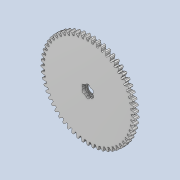
# Autodesk Inventor part: m1z57
Saved by Autodesk Inventor 2020.4 (Build 244396000, 396)
## iProperties
Created: 2021-04-23
Part Number: m1z57
Material: アルミニウム 2014-T4
Document SubType Name: Modeling
Designer: happy
Density: 2.8 g/cm^3
Appearance: サテン
Author: happy
Autodesk Inventor part; units mm, degrees
(part 1 of 2)
ref_plane "YZ Plane" through (0, 0, 0) normal (1, 0, 0) x (0, 1, 0)
ref_plane "XZ Plane" through (0, 0, 0) normal (0, 1, 0) x (-1, 0, 0)
ref_plane "XY Plane" through (0, 0, 0) normal (0, 0, 1) x (1, 0, 0)
sketch "スケッチ1" plane through (0, 0, 0) normal (0, 0, 1) x (1, 0, 0)
  arc A0 (149.0345, 132.7592) -> (148.906, 132.2471) centre (154.9871, 130.993) ccw
  arc A1 (149.29, 133.4958) -> (149.0345, 132.7592) centre (157.261, 130.3183) ccw
  arc A2 (149.7362, 134.4743) -> (149.29, 133.4958) centre (159.5861, 129.3914) ccw
  arc A3 (145.9775, 132.6493) -> (145.9061, 132.1262) centre (152.0883, 131.5486) ccw
  arc A4 (146.1504, 133.4094) -> (145.9775, 132.6493) centre (154.4226, 131.1282) ccw
  arc A5 (146.4863, 134.4312) -> (146.1504, 133.4094) centre (156.8355, 130.4627) ccw
  arc A6 (142.9512, 132.2037) -> (142.9378, 131.676) centre (149.146, 131.782) ccw
  arc A7 (143.0394, 132.9783) -> (142.9512, 132.2037) centre (151.5124, 131.6209) ccw
  arc A8 (143.2609, 134.0308) -> (143.0394, 132.9783) centre (153.9839, 131.2249) ccw
  arc A9 (139.9923, 131.428) -> (140.037, 130.9019) centre (146.1958, 131.6903) ccw
  arc A10 (139.9947, 132.2076) -> (139.9923, 131.428) centre (148.5656, 131.7905) ccw
  arc A11 (140.0991, 133.278) -> (139.9947, 132.2076) centre (151.0656, 131.6688) ccw
  arc A12 (137.1366, 130.3314) -> (137.2389, 129.8135) centre (143.2737, 131.2746) ccw
  arc A13 (137.0533, 131.1065) -> (137.1366, 130.3314) centre (145.618, 131.6349) ccw
  arc A14 (137.0393, 132.182) -> (137.0533, 131.1065) centre (148.1163, 131.789) ccw
  arc A15 (134.4189, 128.9274) -> (134.5776, 128.4239) centre (140.415, 130.5399) ccw
  arc A16 (134.2509, 129.6886) -> (134.4189, 128.9274) centre (142.7055, 131.1559) ccw
  arc A17 (134.1186, 130.756) -> (134.2509, 129.6886) centre (145.1716, 131.5839) ccw
  arc A18 (131.8722, 127.2329) -> (132.0853, 126.7499) centre (137.6545, 129.4953) ccw
  arc A19 (131.6214, 127.971) -> (131.8722, 127.2329) centre (139.8633, 130.3595) ccw
  arc A20 (131.3725, 129.0174) -> (131.6214, 127.971) centre (142.2674, 131.0562) ccw
  arc A21 (129.5273, 125.2685) -> (129.7923, 124.8119) centre (135.0256, 128.1533) ccw
  arc A22 (129.1969, 125.9746) -> (129.5273, 125.2685) centre (137.126, 129.2552) ccw
  arc A23 (128.8344, 126.9872) -> (129.1969, 125.9746) centre (139.4388, 130.2122) ccw
  arc A24 (127.4128, 123.0581) -> (127.7264, 122.6334) centre (132.5604, 126.5302) ccw
  arc A25 (127.0067, 123.7236) -> (127.4128, 123.0581) centre (134.5267, 127.8566) ccw
  arc A26 (126.535, 124.6902) -> (127.0067, 123.7236) centre (136.7203, 129.0621) ccw
  arc A27 (125.5543, 120.6285) -> (125.9126, 120.2409) centre (130.2886, 124.6458) ccw
  arc A28 (125.0774, 121.2453) -> (125.5543, 120.6285) centre (132.0972, 126.1804) ccw
  arc A29 (124.5022, 122.1541) -> (125.0774, 121.2453) centre (134.1448, 127.62) ccw
  arc A30 (123.9743, 118.0092) -> (124.3731, 117.6634) centre (128.238, 122.523) ccw
  arc A31 (123.4325, 118.5698) -> (123.9743, 118.0092) centre (129.8667, 124.2472) ccw
  arc A32 (122.7608, 119.4098) -> (123.4325, 118.5698) centre (131.7435, 125.9033) ccw
  arc A33 (122.692, 115.232) -> (123.1265, 114.9321) centre (126.4333, 120.1874) ccw
  arc A34 (122.0918, 115.7295) -> (122.692, 115.232) centre (127.8625, 122.0803) ccw
  arc A35 (121.3318, 116.4906) -> (122.0918, 115.7295) centre (129.5457, 123.9328) ccw
  arc A36 (121.7231, 112.3306) -> (122.1879, 112.0803) centre (124.8965, 117.6675) ccw
  arc A37 (121.0718, 112.7591) -> (121.7231, 112.3306) centre (126.1087, 119.7061) ccw
  arc A38 (120.2327, 113.4319) -> (121.0718, 112.7591) centre (127.578, 121.7326) ccw
  arc A39 (121.0792, 109.3402) -> (121.5687, 109.1426) centre (123.6463, 114.9938) ccw
  arc A40 (120.3847, 109.6944) -> (121.0792, 109.3402) centre (124.6269, 117.1534) ccw
  arc A41 (119.4767, 110.2709) -> (120.3847, 109.6944) centre (125.8643, 119.3292) ccw
  arc A42 (120.7682, 106.2971) -> (121.2765, 106.1545) centre (122.6977, 112.1988) ccw
  arc A43 (120.0389, 106.5728) -> (120.7682, 106.2971) centre (123.4348, 114.4532) ccw
  arc A44 (119.073, 107.0458) -> (120.0389, 106.5728) centre (124.4253, 116.7519) ccw
  arc A45 (120.7938, 103.2383) -> (121.3147, 103.1525) centre (122.0624, 109.3164) ccw
  arc A46 (120.0387, 103.4321) -> (120.7938, 103.2383) centre (122.547, 111.6382) ccw
  arc A47 (119.0266, 103.796) -> (120.0387, 103.4321) centre (123.2787, 114.0319) ccw
  arc A48 (121.1558, 100.2008) -> (121.683, 100.1728) centre (121.748, 106.3816) ccw
  arc A49 (120.3839, 100.3104) -> (121.1558, 100.2008) centre (121.9743, 108.7427) ccw
  arc A50 (119.3379, 100.5607) -> (120.3839, 100.3104) centre (122.4382, 111.2023) ccw
  arc A51 (121.8497, 97.2216) -> (122.3768, 97.2518) centre (121.7584, 103.4301) ccw
  arc A52 (121.0705, 97.2456) -> (121.8497, 97.2216) centre (121.7236, 105.8017) ccw
  arc A53 (120.0033, 97.3794) -> (121.0705, 97.2456) centre (121.9141, 108.2974) ccw
  arc A54 (122.8671, 94.3369) -> (123.3877, 94.4248) centre (122.0935, 100.4976) ccw
  arc A55 (122.09, 94.2749) -> (122.8671, 94.3369) centre (121.7979, 102.8509) ccw
  arc A56 (121.0146, 94.2905) -> (122.09, 94.2749) centre (121.7127, 105.3525) ccw
  arc A57 (124.1958, 91.5815) -> (124.7035, 91.7262) centre (122.749, 97.6197) ccw
  arc A58 (123.4302, 91.4345) -> (124.1958, 91.5815) centre (122.1964, 99.9263) ccw
  arc A59 (122.3596, 91.3317) -> (123.4302, 91.4345) centre (121.8365, 102.4033) ccw
  arc A60 (125.8194, 88.9891) -> (126.3081, 89.1888) centre (123.7172, 94.8315) ccw
  arc A61 (125.0747, 88.7587) -> (125.8194, 88.9891) centre (122.9142, 97.0633) ccw
  arc A62 (124.0219, 88.5387) -> (125.0747, 88.7587) centre (122.284, 99.4856) ccw
  arc A63 (127.7184, 86.591) -> (128.1822, 86.8432) centre (124.9863, 92.1667) ccw
  arc A64 (127.0035, 86.2801) -> (127.7184, 86.591) centre (123.9426, 94.2965) ccw
  arc A65 (125.9813, 85.9456) -> (127.0035, 86.2801) centre (123.0498, 96.6349) ccw
  arc A66 (129.8697, 84.4163) -> (130.3029, 84.7181) centre (126.5408, 89.6576) ccw
  arc A67 (129.1933, 84.0287) -> (129.8697, 84.4163) centre (125.2691, 91.6598) ccw
  arc A68 (128.2141, 83.5838) -> (129.1933, 84.0287) centre (124.1245, 93.8857) ccw
  arc A69 (132.2472, 82.4915) -> (132.6446, 82.8391) centre (128.3619, 87.3348) ccw
  arc A70 (131.6176, 82.0318) -> (132.2472, 82.4915) centre (126.8777, 89.1849) ccw
  arc A71 (130.6932, 81.4819) -> (131.6176, 82.0318) centre (125.4951, 91.2714) ccw
  arc A72 (134.822, 80.84) -> (135.1787, 81.2291) centre (130.4274, 85.2264) ccw
  arc A73 (134.2467, 80.3138) -> (134.822, 80.84) centre (128.7487, 86.902) ccw
  arc A74 (133.3885, 79.6656) -> (134.2467, 80.3138) centre (127.145, 88.8238) ccw
  arc A75 (137.5628, 79.4817) -> (137.8746, 79.9077) centre (132.7124, 83.3581) ccw
  arc A76 (137.0489, 78.8954) -> (137.5628, 79.4817) centre (130.8595, 84.8389) ccw
  arc A77 (136.2672, 78.1567) -> (137.0489, 78.8954) centre (129.0541, 86.5725) ccw
  arc A78 (140.4364, 78.4331) -> (140.6994, 78.8909) centre (135.189, 81.7524) ccw
  arc A79 (139.9902, 77.7939) -> (140.4364, 78.4331) centre (133.1845, 83.0204) ccw
  arc A80 (139.2945, 76.9737) -> (139.9902, 77.7939) centre (131.1993, 84.5449) ccw
  arc A81 (143.4079, 77.7071) -> (143.619, 78.191) centre (137.8272, 80.429) ccw
  arc A82 (143.0347, 77.0227) -> (143.4079, 77.7071) centre (135.6954, 81.4687) ccw
  arc A83 (142.4335, 76.1309) -> (143.0347, 77.0227) centre (133.5546, 82.7656) ccw
  arc A84 (146.4413, 77.3123) -> (146.5978, 77.8165) centre (140.595, 79.4038) ccw
  arc A85 (146.1456, 76.591) -> (146.4413, 77.3123) centre (138.3618, 80.2027) ccw
  arc A86 (145.6462, 75.6385) -> (146.1456, 76.591) centre (136.0913, 81.2562) ccw
  arc A87 (149.4997, 77.2537) -> (149.5998, 77.772) centre (143.4588, 78.6893) ccw
  arc A88 (149.2852, 76.5042) -> (149.4997, 77.2537) centre (141.1512, 79.2377) ccw
  arc A89 (148.8935, 75.5025) -> (149.2852, 76.5042) centre (138.7786, 80.035) ccw
  arc A90 (152.546, 77.5318) -> (152.5884, 78.0581) centre (146.3838, 78.2942) ccw
  arc A91 (152.4152, 76.7633) -> (152.546, 77.5318) centre (144.0299, 78.5854) ccw
  arc A92 (152.1361, 75.7246) -> (152.4152, 76.7633) centre (141.584, 79.1169) ccw
  arc A93 (155.5431, 78.1434) -> (155.5275, 78.6711) centre (149.3345, 78.2232) ccw
  arc A94 (155.4977, 77.3651) -> (155.5431, 78.1434) centre (146.9629, 78.2537) ccw
  arc A95 (155.3346, 76.3021) -> (155.4977, 77.3651) centre (144.4733, 78.5129) ccw
  arc A96 (158.4549, 79.081) -> (158.3812, 79.6038) centre (152.2752, 78.4773) ccw
  arc A97 (158.4953, 78.3024) -> (158.4549, 79.081) centre (149.9145, 78.2467) ccw
  arc A98 (158.4501, 77.2279) -> (158.4953, 78.3024) centre (147.4116, 78.2305) ccw
  arc A99 (161.2458, 80.3332) -> (161.1151, 80.8447) centre (155.17, 79.0534) ccw
  arc A100 (161.3716, 79.5638) -> (161.2458, 80.3332) centre (152.849, 78.5645) ccw
  arc A101 (161.4449, 78.4908) -> (161.3716, 79.5638) centre (150.3631, 78.273) ccw
  arc A102 (163.882, 81.8848) -> (163.6958, 82.3788) centre (157.9838, 79.9444) ccw
  arc A103 (164.0917, 81.1339) -> (163.882, 81.8848) centre (155.7308, 79.2031) ccw
  arc A104 (164.2826, 80.0755) -> (164.0917, 81.1339) centre (153.292, 78.6399) ccw
  arc A105 (166.3315, 83.717) -> (166.0921, 84.1875) centre (160.6826, 81.1395) ccw
  arc A106 (166.6226, 82.9938) -> (166.3315, 83.717) centre (158.5248, 80.1549) ccw
  arc A107 (166.9287, 81.9627) -> (166.6226, 82.9938) centre (156.1627, 79.3269) ccw
  arc A108 (168.5646, 85.8075) -> (168.2749, 86.2489) centre (163.2335, 82.6243) ccw
  arc A109 (168.9334, 85.1207) -> (168.5646, 85.8075) centre (161.1971, 81.4083) ccw
  arc A110 (169.3512, 84.1296) -> (168.9334, 85.1207) centre (158.9405, 80.3254) ccw
  arc A111 (170.5541, 88.1311) -> (170.2177, 88.5379) centre (165.6056, 84.3807) ccw
  arc A112 (170.9963, 87.489) -> (170.5541, 88.1311) centre (163.7153, 82.948) ccw
  arc A113 (171.5205, 86.5499) -> (170.9963, 87.489) centre (161.5915, 81.6235) ccw
  arc A114 (172.276, 90.6594) -> (171.8968, 91.0267) centre (167.7701, 86.3874) ccw
  arc A115 (172.7861, 90.0698) -> (172.276, 90.6594) centre (166.0489, 84.7555) ccw
  arc A116 (173.4105, 89.1941) -> (172.7861, 90.0698) centre (164.0837, 83.2053) ccw
  arc A117 (173.7093, 93.3617) -> (173.292, 93.6851) centre (169.7007, 88.62) ccw
  arc A118 (174.2812, 92.8319) -> (173.7093, 93.3617) centre (168.1695, 86.8086) ccw
  arc A119 (174.9981, 92.0301) -> (174.2812, 92.8319) centre (166.3867, 85.0517) ccw
  arc A120 (174.8366, 96.2054) -> (174.3863, 96.4809) centre (171.374, 91.0514) ccw
  arc A121 (175.4633, 95.7417) -> (174.8366, 96.2054) centre (170.0513, 89.0826) ccw
  arc A122 (176.2641, 95.0236) -> (175.4633, 95.7417) centre (168.4727, 87.1402) ccw
  arc A123 (175.6443, 99.1558) -> (175.1664, 99.3801) centre (172.7697, 93.6522) ccw
  arc A124 (176.3182, 98.7638) -> (175.6443, 99.1558) centre (171.6716, 91.5498) ccw
  arc A125 (177.1931, 98.1382) -> (176.3182, 98.7638) centre (170.3162, 89.4455) ccw
  arc A126 (176.1225, 102.1771) -> (175.6228, 102.3475) centre (173.8707, 96.3907) ccw
  arc A127 (176.8354, 101.8617) -> (176.1225, 102.1771) centre (173.0106, 94.1803) ccw
  arc A128 (177.7738, 101.3361) -> (176.8354, 101.8617) centre (171.8949, 91.9397) ccw
  arc A129 (176.2654, 105.2327) -> (175.75, 105.3471) centre (174.6639, 99.2337) ccw
  arc A130 (177.0087, 104.9976) -> (176.2654, 105.2327) centre (174.0521, 96.9421) ccw
  arc A131 (177.9992, 104.5785) -> (177.0087, 104.9976) centre (173.1897, 94.5923) ccw
  arc A132 (176.0713, 108.2855) -> (175.5464, 108.3424) centre (175.1394, 102.1467) ccw
  arc A133 (176.8359, 108.1336) -> (176.0713, 108.2855) centre (174.7835, 99.8017) ccw
  arc A134 (177.8665, 107.826) -> (176.8359, 108.1336) centre (174.1848, 97.3713) ccw
  arc A135 (175.5425, 111.2984) -> (175.0146, 111.2973) centre (175.2916, 105.0943) ccw
  arc A136 (176.3192, 111.2315) -> (175.5425, 111.2984) centre (175.1958, 102.7244) ccw
  arc A137 (177.3774, 111.0391) -> (176.3192, 111.2315) centre (174.8681, 100.2429) ccw
  arc A138 (174.6855, 114.2348) -> (174.1609, 114.1756) centre (175.1187, 108.0408) ccw
  arc A139 (175.4649, 114.2538) -> (174.6855, 114.2348) centre (175.2841, 105.6748) ccw
  arc A140 (176.5378, 114.179) -> (175.4649, 114.2538) centre (175.2314, 103.1723) ccw
  arc A141 (173.5107, 117.0592) -> (172.9958, 116.9426) centre (174.6226, 110.9504) ccw
  arc A142 (174.2833, 117.1638) -> (173.5107, 117.0592) centre (175.0474, 108.6169) ccw
  arc A143 (175.3579, 117.2075) -> (174.2833, 117.1638) centre (175.2702, 106.1238) ccw
  arc A144 (172.0323, 119.7371) -> (171.5334, 119.5646) centre (173.8095, 113.7878) ccw
  arc A145 (172.7887, 119.9261) -> (172.0323, 119.7371) centre (174.4884, 111.5151) ccw
  arc A146 (173.852, 120.0877) -> (172.7887, 119.9261) centre (174.9841, 109.0617) ccw
  arc A147 (170.2683, 122.2362) -> (169.7913, 122.0099) centre (172.6892, 116.5185) ccw
  arc A148 (170.9993, 122.5072) -> (170.2683, 122.2362) centre (173.6139, 114.3343) ccw
  arc A149 (172.0384, 122.7849) -> (170.9993, 122.5072) centre (174.3766, 111.9503) ccw
  arc A150 (168.2401, 124.526) -> (167.7909, 124.2486) centre (171.2752, 119.1093) ccw
  arc A151 (168.9368, 124.8758) -> (168.2401, 124.526) centre (172.4347, 117.0402) ccw
  arc A152 (169.939, 125.2661) -> (168.9368, 124.8758) centre (173.455, 114.7545) ccw
  arc A153 (165.9723, 126.5789) -> (165.5563, 126.2537) centre (169.5849, 121.5289) ccw
  arc A154 (166.6263, 127.0032) -> (165.9723, 126.5789) centre (170.9649, 119.5999) ccw
  arc A155 (167.5795, 127.5013) -> (166.6263, 127.0032) centre (172.2304, 117.4404) ccw
  arc A156 (163.4924, 128.3698) -> (163.1147, 128.0008) centre (167.6386, 123.7479) ccw
  arc A157 (164.0957, 128.8635) -> (163.4924, 128.3698) centre (169.2225, 121.9823) ccw
  arc A158 (164.9884, 129.4634) -> (164.0957, 128.8635) centre (170.7179, 119.9752) ccw
  arc A159 (160.8305, 129.877) -> (160.4958, 129.4688) centre (165.46, 125.7393) ccw
  arc A160 (161.3759, 130.434) -> (160.8305, 129.877) centre (167.2285, 124.1587) ccw
  arc A161 (162.1971, 131.1286) -> (161.3759, 130.434) centre (168.9357, 122.3282) ccw
  arc A162 (158.019, 131.0822) -> (157.7312, 130.6397) centre (163.0756, 127.4789) ccw
  arc A163 (158.4998, 131.6959) -> (158.019, 131.0822) centre (165.0072, 126.1025) ccw
  arc A164 (159.2397, 132.4766) -> (158.4998, 131.6959) centre (166.9054, 124.4709) ccw
  arc A165 (155.092, 131.9709) -> (154.8546, 131.4993) centre (160.5143, 128.9457) ccw
  arc A166 (155.5024, 132.6337) -> (155.092, 131.9709) centre (162.5856, 127.7901) ccw
  arc A167 (156.1518, 133.491) -> (155.5024, 132.6337) centre (164.6518, 126.3772) ccw
  arc A168 (152.0848, 132.5318) -> (151.9009, 132.0373) centre (157.8071, 130.1218) ccw
  arc A169 (152.4201, 133.2365) -> (152.0848, 132.5318) centre (159.993, 129.2012) ccw
  arc A170 (152.9711, 134.1596) -> (152.4201, 133.2365) centre (162.202, 128.0241) ccw
  arc A171 (148.0982, 132.2471) -> (147.9697, 132.7592) centre (142.0171, 130.9929) ccw
  arc A172 (147.9697, 132.7592) -> (147.7142, 133.4957) centre (139.7432, 130.3183) ccw
  arc A173 (147.7142, 133.4957) -> (147.2679, 134.4743) centre (137.4181, 129.3914) ccw
  arc A174 (145.1033, 132.0373) -> (144.9192, 132.5321) centre (139.197, 130.1218) ccw
  arc A175 (144.9192, 132.5321) -> (144.5842, 133.2361) centre (137.0111, 129.2011) ccw
  arc A176 (144.5842, 133.2361) -> (144.033, 134.1596) centre (134.8021, 128.0241) ccw
  arc A177 (142.1496, 131.4993) -> (141.9122, 131.9709) centre (136.4899, 128.9457) ccw
  arc A178 (141.9122, 131.9709) -> (141.5018, 132.6337) centre (134.4186, 127.7901) ccw
  arc A179 (141.5018, 132.6337) -> (140.8524, 133.491) centre (132.3524, 126.3772) ccw
  arc A180 (139.273, 130.6397) -> (138.9852, 131.0822) centre (133.9286, 127.4789) ccw
  arc A181 (138.9852, 131.0822) -> (138.5044, 131.6959) centre (131.997, 126.1025) ccw
  arc A182 (138.5044, 131.6959) -> (137.7645, 132.4766) centre (130.0988, 124.4709) ccw
  arc A183 (136.5084, 129.4688) -> (136.1737, 129.877) centre (131.5441, 125.7393) ccw
  arc A184 (136.1737, 129.877) -> (135.6283, 130.434) centre (129.7757, 124.1587) ccw
  arc A185 (135.6283, 130.434) -> (134.8071, 131.1286) centre (128.0685, 122.3282) ccw
  arc A186 (133.8894, 128.0008) -> (133.5118, 128.3698) centre (129.3656, 123.7479) ccw
  arc A187 (133.5118, 128.3698) -> (132.9085, 128.8635) centre (127.7817, 121.9823) ccw
  arc A188 (132.9085, 128.8635) -> (132.0158, 129.4634) centre (126.2863, 119.9752) ccw
  arc A189 (131.4479, 126.2537) -> (131.0319, 126.5789) centre (127.4193, 121.5289) ccw
  arc A190 (131.0319, 126.5789) -> (130.3779, 127.0032) centre (126.0393, 119.5999) ccw
  arc A191 (130.3779, 127.0032) -> (129.4247, 127.5013) centre (124.7737, 117.4403) ccw
  arc A192 (129.2133, 124.2486) -> (128.7641, 124.526) centre (125.7289, 119.1093) ccw
  arc A193 (128.7641, 124.526) -> (128.0674, 124.8758) centre (124.5695, 117.0402) ccw
  arc A194 (128.0674, 124.8758) -> (127.0652, 125.2661) centre (123.5492, 114.7545) ccw
  arc A195 (127.2128, 122.0099) -> (126.7359, 122.2362) centre (124.315, 116.5185) ccw
  arc A196 (126.7359, 122.2362) -> (126.0049, 122.5072) centre (123.3903, 114.3343) ccw
  arc A197 (126.0049, 122.5072) -> (124.9658, 122.7849) centre (122.6276, 111.9503) ccw
  arc A198 (125.4708, 119.5646) -> (124.9719, 119.7371) centre (123.1947, 113.7878) ccw
  arc A199 (124.9719, 119.7371) -> (124.2155, 119.9261) centre (122.5158, 111.5151) ccw
  arc A200 (124.2155, 119.9261) -> (123.1522, 120.0877) centre (122.02, 109.0617) ccw
  arc A201 (124.0084, 116.9426) -> (123.4935, 117.0592) centre (122.3816, 110.9504) ccw
  arc A202 (123.4935, 117.0592) -> (122.7209, 117.1638) centre (121.9568, 108.6169) ccw
  arc A203 (122.7209, 117.1638) -> (121.6463, 117.2075) centre (121.734, 106.1238) ccw
  arc A204 (122.8433, 114.1756) -> (122.3187, 114.2348) centre (121.8855, 108.0408) ccw
  arc A205 (122.3187, 114.2348) -> (121.5393, 114.2538) centre (121.7201, 105.6747) ccw
  arc A206 (121.5393, 114.2538) -> (120.4664, 114.179) centre (121.7728, 103.1723) ccw
  arc A207 (121.9896, 111.2973) -> (121.4617, 111.2984) centre (121.7126, 105.0943) ccw
  arc A208 (121.4617, 111.2984) -> (120.685, 111.2315) centre (121.8084, 102.7244) ccw
  arc A209 (120.685, 111.2315) -> (119.6268, 111.0391) centre (122.1361, 100.2429) ccw
  arc A210 (121.4578, 108.3424) -> (120.9329, 108.2855) centre (121.8648, 102.1467) ccw
  arc A211 (120.9329, 108.2855) -> (120.1683, 108.1336) centre (122.2207, 99.8017) ccw
  arc A212 (120.1683, 108.1336) -> (119.1377, 107.826) centre (122.8194, 97.3713) ccw
  arc A213 (121.2542, 105.3471) -> (120.7388, 105.2327) centre (122.3403, 99.2337) ccw
  arc A214 (120.7388, 105.2327) -> (119.9955, 104.9976) centre (122.9521, 96.9421) ccw
  arc A215 (119.9955, 104.9976) -> (119.005, 104.5785) centre (123.8145, 94.5923) ccw
  arc A216 (121.3814, 102.3475) -> (120.8817, 102.1771) centre (123.1335, 96.3907) ccw
  arc A217 (120.8817, 102.1771) -> (120.1688, 101.8617) centre (123.9936, 94.1803) ccw
  arc A218 (120.1688, 101.8617) -> (119.2304, 101.3361) centre (125.1093, 91.9397) ccw
  arc A219 (121.8378, 99.3801) -> (121.3599, 99.1558) centre (124.2345, 93.6522) ccw
  arc A220 (121.3599, 99.1558) -> (120.686, 98.7638) centre (125.3326, 91.5498) ccw
  arc A221 (120.686, 98.7638) -> (119.8111, 98.1382) centre (126.688, 89.4455) ccw
  arc A222 (122.6179, 96.4809) -> (122.1676, 96.2054) centre (125.6302, 91.0514) ccw
  arc A223 (122.1676, 96.2054) -> (121.5409, 95.7417) centre (126.9529, 89.0826) ccw
  arc A224 (121.5409, 95.7417) -> (120.7401, 95.0236) centre (128.5315, 87.1402) ccw
  arc A225 (123.7122, 93.6851) -> (123.2949, 93.3617) centre (127.3035, 88.62) ccw
  arc A226 (123.2949, 93.3617) -> (122.723, 92.8319) centre (128.8347, 86.8086) ccw
  arc A227 (122.723, 92.8319) -> (122.0061, 92.0301) centre (130.6175, 85.0517) ccw
  arc A228 (125.1074, 91.0267) -> (124.7282, 90.6594) centre (129.2341, 86.3874) ccw
  arc A229 (124.7282, 90.6594) -> (124.218, 90.0698) centre (130.9553, 84.7555) ccw
  arc A230 (124.218, 90.0698) -> (123.5937, 89.1941) centre (132.9205, 83.2053) ccw
  arc A231 (126.7865, 88.5379) -> (126.4501, 88.1311) centre (131.3985, 84.3807) ccw
  arc A232 (126.4501, 88.1311) -> (126.0079, 87.489) centre (133.2889, 82.948) ccw
  arc A233 (126.0079, 87.489) -> (125.4837, 86.5499) centre (135.4127, 81.6235) ccw
  arc A234 (128.7293, 86.2489) -> (128.4396, 85.8076) centre (133.7707, 82.6243) ccw
  arc A235 (128.4396, 85.8076) -> (128.0708, 85.1207) centre (135.8071, 81.4083) ccw
  arc A236 (128.0708, 85.1207) -> (127.653, 84.1296) centre (138.0637, 80.3254) ccw
  arc A237 (130.9121, 84.1875) -> (130.6727, 83.717) centre (136.3216, 81.1395) ccw
  arc A238 (130.6727, 83.717) -> (130.3816, 82.9938) centre (138.4794, 80.1549) ccw
  arc A239 (130.3816, 82.9938) -> (130.0755, 81.9627) centre (140.8415, 79.3269) ccw
  arc A240 (133.3084, 82.3788) -> (133.1222, 81.8848) centre (139.0204, 79.9444) ccw
  arc A241 (133.1222, 81.8848) -> (132.9125, 81.1339) centre (141.2734, 79.2031) ccw
  arc A242 (132.9125, 81.1339) -> (132.7216, 80.0755) centre (143.7122, 78.6399) ccw
  arc A243 (135.8891, 80.8447) -> (135.7584, 80.3332) centre (141.8342, 79.0534) ccw
  arc A244 (135.7584, 80.3332) -> (135.6326, 79.5638) centre (144.1552, 78.5645) ccw
  arc A245 (135.6326, 79.5638) -> (135.5593, 78.4908) centre (146.6411, 78.273) ccw
  arc A246 (138.623, 79.6038) -> (138.5493, 79.081) centre (144.729, 78.4773) ccw
  arc A247 (138.5493, 79.081) -> (138.5089, 78.3024) centre (147.0897, 78.2467) ccw
  arc A248 (138.5089, 78.3024) -> (138.5541, 77.2279) centre (149.5926, 78.2305) ccw
  arc A249 (141.4767, 78.6711) -> (141.4611, 78.1434) centre (147.6697, 78.2232) ccw
  arc A250 (141.4611, 78.1434) -> (141.5065, 77.3651) centre (150.0413, 78.2537) ccw
  arc A251 (141.5065, 77.3651) -> (141.6696, 76.3021) centre (152.5309, 78.5129) ccw
  arc A252 (144.4157, 78.0581) -> (144.4582, 77.5318) centre (150.6204, 78.2942) ccw
  arc A253 (144.4582, 77.5318) -> (144.589, 76.7633) centre (152.9743, 78.5854) ccw
  arc A254 (144.589, 76.7633) -> (144.8681, 75.7246) centre (155.4202, 79.1169) ccw
  arc A255 (147.4044, 77.772) -> (147.5045, 77.2537) centre (153.5454, 78.6893) ccw
  arc A256 (147.5045, 77.2537) -> (147.719, 76.5042) centre (155.853, 79.2377) ccw
  arc A257 (147.719, 76.5042) -> (148.1107, 75.5025) centre (158.2256, 80.035) ccw
  arc A258 (150.4063, 77.8165) -> (150.5629, 77.3123) centre (156.4092, 79.4038) ccw
  arc A259 (150.5629, 77.3123) -> (150.8585, 76.591) centre (158.6424, 80.2027) ccw
  arc A260 (150.8585, 76.591) -> (151.358, 75.6385) centre (160.9129, 81.2562) ccw
  arc A261 (153.3852, 78.191) -> (153.5962, 77.7071) centre (159.177, 80.429) ccw
  arc A262 (153.5962, 77.7071) -> (153.9695, 77.0227) centre (161.3088, 81.4687) ccw
  arc A263 (153.9695, 77.0227) -> (154.5707, 76.1309) centre (163.4496, 82.7656) ccw
  arc A264 (156.3048, 78.8909) -> (156.5678, 78.4331) centre (161.8152, 81.7524) ccw
  arc A265 (156.5678, 78.4331) -> (157.014, 77.7939) centre (163.8197, 83.0204) ccw
  arc A266 (157.014, 77.7939) -> (157.7097, 76.9737) centre (165.8049, 84.5449) ccw
  arc A267 (159.1296, 79.9077) -> (159.4414, 79.4817) centre (164.2918, 83.3581) ccw
  arc A268 (159.4414, 79.4817) -> (159.9553, 78.8954) centre (166.1447, 84.8389) ccw
  arc A269 (159.9553, 78.8954) -> (160.737, 78.1567) centre (167.9501, 86.5725) ccw
  arc A270 (161.8255, 81.2291) -> (162.1822, 80.84) centre (166.5768, 85.2264) ccw
  arc A271 (162.1822, 80.84) -> (162.7575, 80.3138) centre (168.2555, 86.902) ccw
  arc A272 (162.7575, 80.3138) -> (163.6157, 79.6656) centre (169.8592, 88.8238) ccw
  arc A273 (164.3596, 82.8391) -> (164.757, 82.4915) centre (168.6423, 87.3348) ccw
  arc A274 (164.757, 82.4915) -> (165.3866, 82.0318) centre (170.1265, 89.1849) ccw
  arc A275 (165.3866, 82.0318) -> (166.311, 81.4819) centre (171.5091, 91.2714) ccw
  arc A276 (166.7013, 84.7181) -> (167.1345, 84.4163) centre (170.4634, 89.6576) ccw
  arc A277 (167.1345, 84.4163) -> (167.8108, 84.0287) centre (171.7351, 91.6598) ccw
  arc A278 (167.8108, 84.0287) -> (168.7901, 83.5838) centre (172.8797, 93.8857) ccw
  arc A279 (168.822, 86.8432) -> (169.2858, 86.591) centre (172.0179, 92.1667) ccw
  arc A280 (169.2858, 86.591) -> (170.0007, 86.2801) centre (173.0616, 94.2966) ccw
  arc A281 (170.0007, 86.2801) -> (171.0229, 85.9456) centre (173.9544, 96.6349) ccw
  arc A282 (170.6961, 89.1888) -> (171.1848, 88.9891) centre (173.287, 94.8315) ccw
  arc A283 (171.1848, 88.9891) -> (171.9295, 88.7587) centre (174.09, 97.0633) ccw
  arc A284 (171.9295, 88.7587) -> (172.9823, 88.5387) centre (174.7202, 99.4856) ccw
  arc A285 (172.3007, 91.7262) -> (172.8084, 91.5815) centre (174.2552, 97.6197) ccw
  arc A286 (172.8084, 91.5815) -> (173.574, 91.4345) centre (174.8078, 99.9263) ccw
  arc A287 (173.574, 91.4345) -> (174.6446, 91.3317) centre (175.1677, 102.4033) ccw
  arc A288 (173.6165, 94.4248) -> (174.1371, 94.3369) centre (174.9107, 100.4976) ccw
  arc A289 (174.1371, 94.3369) -> (174.9142, 94.275) centre (175.2063, 102.8509) ccw
  arc A290 (174.9142, 94.275) -> (175.9896, 94.2905) centre (175.2915, 105.3525) ccw
  arc A291 (174.6274, 97.2518) -> (175.1545, 97.2216) centre (175.2458, 103.4301) ccw
  arc A292 (175.1545, 97.2216) -> (175.9337, 97.2456) centre (175.2806, 105.8017) ccw
  arc A293 (175.9337, 97.2456) -> (177.0009, 97.3794) centre (175.0901, 108.2974) ccw
  arc A294 (175.3212, 100.1729) -> (175.8484, 100.2008) centre (175.2562, 106.3816) ccw
  arc A295 (175.8484, 100.2008) -> (176.6203, 100.3104) centre (175.0299, 108.7427) ccw
  arc A296 (176.6203, 100.3104) -> (177.6663, 100.5607) centre (174.566, 111.2023) ccw
  arc A297 (175.6895, 103.1525) -> (176.2104, 103.2383) centre (174.9418, 109.3164) ccw
  arc A298 (176.2104, 103.2383) -> (176.9655, 103.4321) centre (174.4572, 111.6382) ccw
  arc A299 (176.9655, 103.4321) -> (177.9776, 103.796) centre (173.7255, 114.0319) ccw
  arc A300 (175.7277, 106.1545) -> (176.236, 106.2971) centre (174.3065, 112.1988) ccw
  arc A301 (176.236, 106.2971) -> (176.9653, 106.5728) centre (173.5694, 114.4532) ccw
  arc A302 (176.9653, 106.5728) -> (177.9312, 107.0458) centre (172.5788, 116.7519) ccw
  arc A303 (175.4355, 109.1426) -> (175.925, 109.3402) centre (173.3579, 114.9938) ccw
  arc A304 (175.925, 109.3402) -> (176.6195, 109.6944) centre (172.3773, 117.1534) ccw
  arc A305 (176.6195, 109.6944) -> (177.5275, 110.2709) centre (171.1399, 119.3292) ccw
  arc A306 (174.8163, 112.0803) -> (175.2811, 112.3306) centre (172.1077, 117.6675) ccw
  arc A307 (175.2811, 112.3306) -> (175.9324, 112.7591) centre (170.8954, 119.7062) ccw
  arc A308 (175.9324, 112.7591) -> (176.7715, 113.4319) centre (169.4262, 121.7326) ccw
  arc A309 (173.8777, 114.9321) -> (174.3122, 115.232) centre (170.5709, 120.1874) ccw
  arc A310 (174.3122, 115.232) -> (174.9124, 115.7295) centre (169.1417, 122.0803) ccw
  arc A311 (174.9124, 115.7295) -> (175.6723, 116.4906) centre (167.4585, 123.9328) ccw
  arc A312 (172.6311, 117.6634) -> (173.0299, 118.0092) centre (168.7662, 122.523) ccw
  arc A313 (173.0299, 118.0092) -> (173.5717, 118.5698) centre (167.1375, 124.2472) ccw
  arc A314 (173.5717, 118.5698) -> (174.2434, 119.4098) centre (165.2607, 125.9033) ccw
  arc A315 (171.0916, 120.2409) -> (171.4499, 120.6285) centre (166.7155, 124.6458) ccw
  arc A316 (171.4499, 120.6285) -> (171.9268, 121.2453) centre (164.907, 126.1804) ccw
  arc A317 (171.9268, 121.2453) -> (172.502, 122.1541) centre (162.8594, 127.62) ccw
  arc A318 (169.2778, 122.6334) -> (169.5914, 123.0581) centre (164.4438, 126.5302) ccw
  arc A319 (169.5914, 123.0581) -> (169.9975, 123.7236) centre (162.4774, 127.8566) ccw
  arc A320 (169.9975, 123.7236) -> (170.4692, 124.6902) centre (160.2839, 129.0621) ccw
  arc A321 (167.2119, 124.8119) -> (167.4768, 125.2685) centre (161.9785, 128.1533) ccw
  arc A322 (167.4768, 125.2685) -> (167.8073, 125.9746) centre (159.8782, 129.2552) ccw
  arc A323 (167.8073, 125.9746) -> (168.1698, 126.9872) centre (157.5654, 130.2122) ccw
  arc A324 (164.9189, 126.7499) -> (165.132, 127.2329) centre (159.3497, 129.4953) ccw
  arc A325 (165.132, 127.2329) -> (165.3828, 127.971) centre (157.1409, 130.3595) ccw
  arc A326 (165.3828, 127.971) -> (165.6317, 129.0174) centre (154.7368, 131.0562) ccw
  arc A327 (162.4266, 128.4239) -> (162.5852, 128.9274) centre (156.5892, 130.5399) ccw
  arc A328 (162.5852, 128.9274) -> (162.7533, 129.6886) centre (154.2987, 131.1559) ccw
  arc A329 (162.7533, 129.6886) -> (162.8856, 130.756) centre (151.8326, 131.5839) ccw
  arc A330 (159.7653, 129.8135) -> (159.8676, 130.3314) centre (153.7305, 131.2746) ccw
  arc A331 (159.8676, 130.3314) -> (159.9509, 131.1065) centre (151.3862, 131.6349) ccw
  arc A332 (159.9509, 131.1065) -> (159.9649, 132.182) centre (148.8879, 131.789) ccw
  arc A333 (156.9672, 130.9019) -> (157.0119, 131.428) centre (150.8084, 131.6903) ccw
  arc A334 (157.0119, 131.428) -> (157.0094, 132.2076) centre (148.4386, 131.7905) ccw
  arc A335 (157.0094, 132.2076) -> (156.9051, 133.278) centre (145.9386, 131.6688) ccw
  arc A336 (154.0664, 131.676) -> (154.053, 132.2037) centre (147.8582, 131.782) ccw
  arc A337 (154.053, 132.2037) -> (153.9648, 132.9783) centre (145.4918, 131.6209) ccw
  arc A338 (153.9648, 132.9783) -> (153.7433, 134.0308) centre (143.0203, 131.2249) ccw
  arc A339 (151.098, 132.1262) -> (151.0266, 132.6493) centre (144.9158, 131.5487) ccw
  arc A340 (151.0266, 132.6493) -> (150.8537, 133.4095) centre (142.5815, 131.1282) ccw
  arc A341 (150.8537, 133.4095) -> (150.5178, 134.4312) centre (140.1686, 130.4628) ccw
  arc A342 (148.906, 132.2471) -> (148.0982, 132.2471) centre (148.5021, 105) ccw
  arc A343 (145.9061, 132.1262) -> (145.1033, 132.0373) centre (148.5021, 105) ccw
  arc A344 (142.9378, 131.676) -> (142.1496, 131.4993) centre (148.5021, 105) ccw
  arc A345 (140.037, 130.9019) -> (139.273, 130.6397) centre (148.5021, 105) ccw
  arc A346 (137.2389, 129.8135) -> (136.5084, 129.4688) centre (148.5021, 105) ccw
  arc A347 (134.5776, 128.4239) -> (133.8894, 128.0008) centre (148.5021, 105) ccw
  arc A348 (132.0853, 126.7499) -> (131.4479, 126.2537) centre (148.5021, 105) ccw
  arc A349 (129.7923, 124.8119) -> (129.2133, 124.2486) centre (148.5021, 105) ccw
  arc A350 (127.7264, 122.6334) -> (127.2128, 122.0099) centre (148.5021, 105) ccw
  arc A351 (125.9126, 120.2409) -> (125.4708, 119.5646) centre (148.5021, 105) ccw
  arc A352 (124.3731, 117.6634) -> (124.0084, 116.9426) centre (148.5021, 105) ccw
  arc A353 (123.1265, 114.9321) -> (122.8433, 114.1756) centre (148.5021, 105) ccw
  arc A354 (122.1879, 112.0803) -> (121.9896, 111.2973) centre (148.5021, 105) ccw
  arc A355 (121.5687, 109.1426) -> (121.4578, 108.3424) centre (148.5021, 105) ccw
  arc A356 (121.2765, 106.1545) -> (121.2542, 105.3471) centre (148.5021, 105) ccw
  arc A357 (121.3147, 103.1525) -> (121.3814, 102.3475) centre (148.5021, 105) ccw
  arc A358 (121.683, 100.1728) -> (121.8378, 99.3801) centre (148.5021, 105) ccw
  arc A359 (122.3768, 97.2518) -> (122.6179, 96.4809) centre (148.5021, 105) ccw
  arc A360 (123.3877, 94.4248) -> (123.7122, 93.6851) centre (148.5021, 105) ccw
  arc A361 (124.7035, 91.7262) -> (125.1074, 91.0267) centre (148.5021, 105) ccw
  arc A362 (126.3081, 89.1888) -> (126.7865, 88.5379) centre (148.5021, 105) ccw
  arc A363 (128.1822, 86.8432) -> (128.7293, 86.2489) centre (148.5021, 105) ccw
  arc A364 (130.3029, 84.7181) -> (130.9121, 84.1875) centre (148.5021, 105) ccw
  arc A365 (132.6446, 82.8391) -> (133.3084, 82.3788) centre (148.5021, 105) ccw
  arc A366 (135.1787, 81.2291) -> (135.8891, 80.8447) centre (148.5021, 105) ccw
  arc A367 (137.8746, 79.9077) -> (138.623, 79.6038) centre (148.5021, 105) ccw
  arc A368 (140.6994, 78.8909) -> (141.4767, 78.6711) centre (148.5021, 105) ccw
  arc A369 (143.619, 78.191) -> (144.4157, 78.0581) centre (148.5021, 105) ccw
  arc A370 (146.5978, 77.8165) -> (147.4044, 77.772) centre (148.5021, 105) ccw
  arc A371 (149.5998, 77.772) -> (150.4063, 77.8165) centre (148.5021, 105) ccw
  arc A372 (152.5884, 78.0581) -> (153.3852, 78.191) centre (148.5021, 105) ccw
  arc A373 (155.5275, 78.6711) -> (156.3048, 78.8909) centre (148.5021, 105) ccw
  arc A374 (158.3812, 79.6038) -> (159.1296, 79.9077) centre (148.5021, 105) ccw
  arc A375 (161.1151, 80.8447) -> (161.8255, 81.2291) centre (148.5021, 105) ccw
  arc A376 (163.6958, 82.3788) -> (164.3596, 82.8391) centre (148.5021, 105) ccw
  arc A377 (166.0921, 84.1875) -> (166.7013, 84.7181) centre (148.5021, 105) ccw
  arc A378 (168.2749, 86.2489) -> (168.822, 86.8432) centre (148.5021, 105) ccw
  arc A379 (170.2177, 88.5379) -> (170.6961, 89.1888) centre (148.5021, 105) ccw
  arc A380 (171.8968, 91.0267) -> (172.3007, 91.7262) centre (148.5021, 105) ccw
  arc A381 (173.292, 93.6851) -> (173.6165, 94.4248) centre (148.5021, 105) ccw
  arc A382 (174.3863, 96.4809) -> (174.6274, 97.2518) centre (148.5021, 105) ccw
  arc A383 (175.1664, 99.3801) -> (175.3212, 100.1729) centre (148.5021, 105) ccw
  arc A384 (175.6228, 102.3475) -> (175.6895, 103.1525) centre (148.5021, 105) ccw
  arc A385 (175.75, 105.3471) -> (175.7277, 106.1545) centre (148.5021, 105) ccw
  arc A386 (175.5464, 108.3424) -> (175.4355, 109.1426) centre (148.5021, 105) ccw
  arc A387 (175.0146, 111.2973) -> (174.8163, 112.0803) centre (148.5021, 105) ccw
  arc A388 (174.1609, 114.1756) -> (173.8777, 114.9321) centre (148.5021, 105) ccw
  arc A389 (172.9958, 116.9426) -> (172.6311, 117.6634) centre (148.5021, 105) ccw
  arc A390 (171.5334, 119.5646) -> (171.0916, 120.2409) centre (148.5021, 105) ccw
  arc A391 (169.7913, 122.0099) -> (169.2778, 122.6334) centre (148.5021, 105) ccw
  arc A392 (167.7909, 124.2486) -> (167.2119, 124.8119) centre (148.5021, 105) ccw
  arc A393 (165.5563, 126.2537) -> (164.9189, 126.7499) centre (148.5021, 105) ccw
  arc A394 (163.1147, 128.0008) -> (162.4266, 128.4239) centre (148.5021, 105) ccw
  arc A395 (160.4958, 129.4688) -> (159.7653, 129.8135) centre (148.5021, 105) ccw
  arc A396 (157.7312, 130.6397) -> (156.9672, 130.9019) centre (148.5021, 105) ccw
  arc A397 (154.8546, 131.4993) -> (154.0664, 131.676) centre (148.5021, 105) ccw
  arc A398 (151.9009, 132.0373) -> (151.098, 132.1262) centre (148.5021, 105) ccw
  arc A399 (147.2679, 134.4743) -> (146.4863, 134.4312) centre (148.5021, 105) ccw
  arc A400 (144.033, 134.1596) -> (143.2609, 134.0308) centre (148.5021, 105) ccw
  arc A401 (140.8524, 133.491) -> (140.0991, 133.278) centre (148.5021, 105) ccw
  arc A402 (137.7645, 132.4766) -> (137.0393, 132.182) centre (148.5021, 105) ccw
  arc A403 (134.8071, 131.1286) -> (134.1186, 130.756) centre (148.5021, 105) ccw
  arc A404 (132.0158, 129.4634) -> (131.3725, 129.0174) centre (148.5021, 105) ccw
  arc A405 (129.4247, 127.5013) -> (128.8344, 126.9872) centre (148.5021, 105) ccw
  arc A406 (127.0652, 125.2661) -> (126.535, 124.6902) centre (148.5021, 105) ccw
  arc A407 (124.9658, 122.7849) -> (124.5022, 122.1541) centre (148.5021, 105) ccw
  arc A408 (123.1522, 120.0877) -> (122.7608, 119.4098) centre (148.5021, 105) ccw
  arc A409 (121.6463, 117.2075) -> (121.3318, 116.4906) centre (148.5021, 105) ccw
  arc A410 (120.4664, 114.179) -> (120.2327, 113.4319) centre (148.5021, 105) ccw
  arc A411 (119.6268, 111.0391) -> (119.4767, 110.2709) centre (148.5021, 105) ccw
  arc A412 (119.1377, 107.826) -> (119.073, 107.0458) centre (148.5021, 105) ccw
  arc A413 (119.005, 104.5785) -> (119.0266, 103.796) centre (148.5021, 105) ccw
  arc A414 (119.2304, 101.3361) -> (119.3379, 100.5607) centre (148.5021, 105) ccw
  arc A415 (119.8111, 98.1382) -> (120.0033, 97.3794) centre (148.5021, 105) ccw
  arc A416 (120.7401, 95.0236) -> (121.0146, 94.2905) centre (148.5021, 105) ccw
  arc A417 (122.0061, 92.0301) -> (122.3596, 91.3317) centre (148.5021, 105) ccw
  arc A418 (123.5937, 89.1941) -> (124.0219, 88.5387) centre (148.5021, 105) ccw
  arc A419 (125.4837, 86.5499) -> (125.9813, 85.9456) centre (148.5021, 105) ccw
  arc A420 (127.653, 84.1296) -> (128.2141, 83.5838) centre (148.5021, 105) ccw
  arc A421 (130.0755, 81.9627) -> (130.6932, 81.4819) centre (148.5021, 105) ccw
  arc A422 (132.7216, 80.0755) -> (133.3885, 79.6656) centre (148.5021, 105) ccw
  arc A423 (135.5593, 78.4908) -> (136.2672, 78.1567) centre (148.5021, 105) ccw
  arc A424 (138.5541, 77.2279) -> (139.2945, 76.9737) centre (148.5021, 105) ccw
  arc A425 (141.6696, 76.3021) -> (142.4335, 76.1309) centre (148.5021, 105) ccw
  arc A426 (144.8681, 75.7246) -> (145.6462, 75.6385) centre (148.5021, 105) ccw
  arc A427 (148.1107, 75.5025) -> (148.8935, 75.5025) centre (148.5021, 105) ccw
  arc A428 (151.358, 75.6385) -> (152.1361, 75.7246) centre (148.5021, 105) ccw
  arc A429 (154.5707, 76.1309) -> (155.3346, 76.3021) centre (148.5021, 105) ccw
  arc A430 (157.7097, 76.9737) -> (158.4501, 77.2279) centre (148.5021, 105) ccw
  arc A431 (160.737, 78.1567) -> (161.4449, 78.4908) centre (148.5021, 105) ccw
  arc A432 (163.6157, 79.6656) -> (164.2826, 80.0755) centre (148.5021, 105) ccw
  arc A433 (166.311, 81.4819) -> (166.9287, 81.9627) centre (148.5021, 105) ccw
  arc A434 (168.7901, 83.5838) -> (169.3512, 84.1296) centre (148.5021, 105) ccw
  arc A435 (171.0229, 85.9456) -> (171.5205, 86.5499) centre (148.5021, 105) ccw
  arc A436 (172.9823, 88.5387) -> (173.4105, 89.1941) centre (148.5021, 105) ccw
  arc A437 (174.6446, 91.3317) -> (174.9981, 92.0301) centre (148.5021, 105) ccw
  arc A438 (175.9896, 94.2905) -> (176.2641, 95.0236) centre (148.5021, 105) ccw
  arc A439 (177.0009, 97.3794) -> (177.1931, 98.1382) centre (148.5021, 105) ccw
  arc A440 (177.6663, 100.5607) -> (177.7738, 101.3361) centre (148.5021, 105) ccw
  arc A441 (177.9776, 103.796) -> (177.9992, 104.5785) centre (148.5021, 105) ccw
  arc A442 (177.9312, 107.0458) -> (177.8665, 107.826) centre (148.5021, 105) ccw
  arc A443 (177.5275, 110.2709) -> (177.3774, 111.0391) centre (148.5021, 105) ccw
  arc A444 (176.7715, 113.4319) -> (176.5378, 114.179) centre (148.5021, 105) ccw
  arc A445 (175.6723, 116.4906) -> (175.3579, 117.2075) centre (148.5021, 105) ccw
  arc A446 (174.2434, 119.4098) -> (173.852, 120.0877) centre (148.5021, 105) ccw
  arc A447 (172.502, 122.1541) -> (172.0384, 122.7849) centre (148.5021, 105) ccw
  arc A448 (170.4692, 124.6902) -> (169.939, 125.2661) centre (148.5021, 105) ccw
  arc A449 (168.1698, 126.9872) -> (167.5795, 127.5013) centre (148.5021, 105) ccw
  arc A450 (165.6317, 129.0174) -> (164.9884, 129.4634) centre (148.5021, 105) ccw
  arc A451 (162.8856, 130.756) -> (162.1971, 131.1286) centre (148.5021, 105) ccw
  arc A452 (159.9649, 132.182) -> (159.2397, 132.4766) centre (148.5021, 105) ccw
  arc A453 (156.9051, 133.278) -> (156.1518, 133.491) centre (148.5021, 105) ccw
  arc A454 (153.7433, 134.0308) -> (152.9711, 134.1596) centre (148.5021, 105) ccw
  arc A455 (150.5178, 134.4312) -> (149.7362, 134.4743) centre (148.5021, 105) ccw
  line L0 (117, 105) -> (180, 105)
  line L1 (148.5021, 73.5001) -> (148.5021, 136.5001)
  line L2 (198, 134.5001) -> (268, 134.5001)
  line L3 (198, 126.5001) -> (268, 126.5001)
  line L4 (198, 118.5001) -> (268, 118.5001)
  line L5 (198, 110.5001) -> (268, 110.5001)
  line L6 (198, 102.5001) -> (268, 102.5001)
  line L7 (198, 94.5001) -> (268, 94.5001)
  line L8 (198, 86.5001) -> (268, 86.5001)
  line L9 (198, 78.5001) -> (268, 78.5001)
  line L10 (198, 70.5001) -> (268, 70.5001)
  line L11 (198, 62.5001) -> (268, 62.5001)
  line L12 (198, 54.5001) -> (268, 54.5001)
  line L13 (198, 46.5001) -> (268, 46.5001)
  line L14 (198, 38.5001) -> (268, 38.5001)
  line L15 (198, 134.5001) -> (198, 38.5001)
  line L16 (268, 134.5001) -> (268, 38.5001)
  line L17 (233, 126.5001) -> (233, 38.5001)
  circle A456 centre (148.5021, 105) radius 2.025
  point P0 (0, 0)
  point P1 (204, 128.5)
  point P2 (206.5, 120.5)
  point P3 (206.5, 112.5)
  point P4 (204, 104.5)
  point P5 (206.5, 96.5)
  point P6 (201.5, 88.5)
  point P7 (204, 80.5)
  point P8 (204, 72.5)
  point P9 (204, 64.5)
  point P10 (206.5, 56.5)
  point P11 (206.5, 48.5)
  point P12 (204, 40.5)
  point P13 (234, 120.5)
  point P14 (249, 112.5)
  point P15 (250.25, 104.5)
  point P16 (246.5, 96.5)
  point P17 (249, 88.5)
  point P18 (242.75, 80.5)
  point P19 (249, 72.5)
  point P20 (246.5, 64.5)
  point P21 (244, 56.5)
  point P22 (251.5, 48.5)
  point P23 (251.5, 40.5)
  point P24 (149.5, 150)
  point P25 (149.5, 144)
  point P26 (165.6875, 150)
  point P27 (167.8125, 144)
  dimension "d0" = 4.05
  constraints: 684 point on circle, 396 equal radius, 343 centre point, 230 tangent, 60 horizontal, 32 end point, 13 parallel, 2 horizontal alignment, 2 midpoint, 2 perpendicular, 1 vertical, 1540 other
  measures "d0" diameter of A456
extrude "押し出し1" add sketch "スケッチ1" along normal blind 2.8 contours A1 A2 A455 A341 A340 A339 A398 A168 A169 A170 A454 A338 A337 A336 A397 A165 A166 A167 A453 A335 A334 A333 A396 A162 A163 A164 A452 A332 A331 A330 A395 A159 A160 A161 A451 A329 A328 A327 A394 A156 A157 A158 A450 A326 A325 A324 A393 A153 A154 A155 A449 A323 A322 A321 A392 A150 A151 A152 A448 A320 A319 A318 A391 A147 A148 A149 A447 A317 A316 A315 A390 A144 A145 A146 A446 A314 A313 A312 A389 A141 A142 A143 A445 A311 A310 A309 A388 A138 A139 A140 A444 A308 A307 A306 A387 A135 A136 A137 A443 A305 A304 A303 A386 A132 A133 A134 A442 A302 A301 A300 A385 A129 A130 L0 A456 L1 A342 A0 | L1 A456 L0 A214 A213 A356 A42 A43 A44 A412 A212 A211 A210 A355 A39 A40 A41 A411 A209 A208 A207 A354 A36 A37 A38 A410 A206 A205 A204 A353 A33 A34 A35 A409 A203 A202 A201 A352 A30 A31 A32 A408 A200 A199 A198 A351 A27 A28 A29 A407 A197 A196 A195 A350 A24 A25 A26 A406 A194 A193 A192 A349 A21 A22 A23 A405 A191 A190 A189 A348 A18 A19 A20 A404 A188 A187 A186 A347 A15 A16 A17 A403 A185 A184 A183 A346 A12 A13 A14 A402 A182 A181 A180 A345 A9 A10 A11 A401 A179 A178 A177 A344 A6 A7 A8 A400 A176 A175 A174 A343 A3 A4 A5 A399 A173 A172 A171 A342 | L0 A130 A131 A441 A299 A298 A297 A384 A126 A127 A128 A440 A296 A295 A294 A383 A123 A124 A125 A439 A293 A292 A291 A382 A120 A121 A122 A438 A290 A289 A288 A381 A117 A118 A119 A437 A287 A286 A285 A380 A114 A115 A116 A436 A284 A283 A282 A379 A111 A112 A113 A435 A281 A280 A279 A378 A108 A109 A110 A434 A278 A277 A276 A377 A105 A106 A107 A433 A275 A274 A273 A376 A102 A103 A104 A432 A272 A271 A270 A375 A99 A100 A101 A431 A269 A268 A267 A374 A96 A97 A98 A430 A266 A265 A264 A373 A93 A94 A95 A429 A263 A262 A261 A372 A90 A91 A92 A428 A260 A259 A258 A371 A87 A88 A89 A427 L1 A456 | A456 L1 A427 A257 A256 A255 A370 A84 A85 A86 A426 A254 A253 A252 A369 A81 A82 A83 A425 A251 A250 A249 A368 A78 A79 A80 A424 A248 A247 A246 A367 A75 A76 A77 A423 A245 A244 A243 A366 A72 A73 A74 A422 A242 A241 A240 A365 A69 A70 A71 A421 A239 A238 A237 A364 A66 A67 A68 A420 A236 A235 A234 A363 A63 A64 A65 A419 A233 A232 A231 A362 A60 A61 A62 A418 A230 A229 A228 A361 A57 A58 A59 A417 A227 A226 A225 A360 A54 A55 A56 A416 A224 A223 A222 A359 A51 A52 A53 A415 A221 A220 A219 A358 A48 A49 A50 A414 A218 A217 A216 A357 A45 A46 A47 A413 A215 A214 L0